Autodesk Inventor part; units mm, degrees
(part 3 of 3)
sketch "Sketch8" plane through (0, 0, 0) normal (0, 0, 1) x (1, 0, 0)
  line L0 (6.1983, 26.6612) -> (5.4238, 26.6612) construction
  line L1 (6.1983, 14.8446) -> (6.1983, 26.6612) projected
  line L2 (6.1293, 14.2121) -> (6.1983, 14.8446) construction
  line L3 (5.9709, 13.7973) -> (6.1293, 14.2121) construction
  line L4 (5.9268, 13.7518) -> (5.9709, 13.7973) construction
  line L5 (5.8813, 13.7077) -> (5.9268, 13.7518) construction
  line L6 (5.4417, 13.5533) -> (5.8813, 13.7077) construction
  line L7 (4.7582, 13.4872) -> (5.4417, 13.5533) construction
  line L8 (3.0618, 13.4872) -> (4.7582, 13.4872) projected
  line L9 (3.0618, 11.5607) -> (3.0618, 13.4872) projected
  line L10 (12.9024, 11.5607) -> (3.0618, 11.5607) projected
  line L11 (12.9024, 13.4872) -> (12.9024, 11.5607) projected
  line L12 (11.2267, 13.4872) -> (12.9024, 13.4872) projected
  line L13 (10.5363, 13.5547) -> (11.2267, 13.4872) construction
  line L14 (10.0898, 13.7132) -> (10.5363, 13.5547) construction
  line L15 (10.0444, 13.7587) -> (10.0898, 13.7132) construction
  line L16 (9.9975, 13.8041) -> (10.0444, 13.7587) construction
  line L17 (9.8349, 14.2189) -> (9.9975, 13.8041) construction
  line L18 (9.766, 14.8473) -> (9.8349, 14.2189) construction
  line L19 (9.766, 26.6612) -> (9.766, 14.8473)
  line L20 (10.5736, 26.6612) -> (9.766, 26.6612) construction
  line L21 (11.8854, 26.3526) -> (10.5736, 26.6612) construction
  line L22 (12.9327, 25.6333) -> (11.8854, 26.3526) construction
  line L23 (13.0871, 25.4265) -> (12.9327, 25.6333) construction
  line L24 (13.2414, 25.2212) -> (13.0871, 25.4265) construction
  line L25 (13.7871, 23.828) -> (13.2414, 25.2212) construction
  line L26 (14.0338, 21.9483) -> (13.7871, 23.828) construction
  line L27 (14.0379, 21.4991) -> (14.0338, 21.9483) construction
  line L28 (15.9768, 21.4991) -> (14.0379, 21.4991)
  line L29 (15.9768, 28.5255) -> (15.9768, 21.4991)
  line L30 (0, 28.5255) -> (15.9768, 28.5255) projected
  line L31 (0, 21.4988) -> (0, 28.5255) projected
  line L32 (1.9389, 21.4988) -> (0, 21.4988) projected
  line L33 (1.9444, 21.9535) -> (1.9389, 21.4988) construction
  line L34 (2.198, 23.8497) -> (1.9444, 21.9535) construction
  line L35 (2.7478, 25.2415) -> (2.198, 23.8497) construction
  line L36 (2.9022, 25.4442) -> (2.7478, 25.2415) construction
  line L37 (3.0565, 25.6467) -> (2.9022, 25.4442) construction
  line L38 (4.1051, 26.3565) -> (3.0565, 25.6467) construction
  line L39 (5.4238, 26.6612) -> (4.1051, 26.3565) construction
  line L40 (1.9444, 21.9535) -> (1.9389, 21.4988) construction
  line L41 (2.198, 23.8497) -> (1.9444, 21.9535) construction
  line L42 (2.7478, 25.2415) -> (2.198, 23.8497) construction
  line L43 (4.1051, 26.3565) -> (3.0565, 25.6467) construction
  line L44 (5.4238, 26.6612) -> (4.1051, 26.3565) construction
  line L45 (6.1983, 26.6612) -> (5.4238, 26.6612) construction
  line L46 (11.8854, 26.3526) -> (10.5736, 26.6612) construction
  line L47 (10.5736, 26.6612) -> (9.766, 26.6612) construction
  line L48 (12.9327, 25.6333) -> (11.8854, 26.3526) construction
  line L49 (13.7871, 23.828) -> (13.2414, 25.2212) construction
  line L50 (14.0338, 21.9483) -> (13.7871, 23.828) construction
  line L51 (14.0379, 21.4991) -> (14.0338, 21.9483) construction
  line L52 (6.1293, 14.2121) -> (6.1983, 14.8446) construction
  line L53 (5.9709, 13.7973) -> (6.1293, 14.2121) construction
  line L54 (5.4417, 13.5533) -> (5.8813, 13.7077) construction
  line L55 (4.7582, 13.4872) -> (5.4417, 13.5533) construction
  line L56 (10.5363, 13.5547) -> (11.2267, 13.4872) construction
  line L57 (10.0898, 13.7132) -> (10.5363, 13.5547) construction
  line L58 (10.0444, 13.7587) -> (10.0898, 13.7132) construction
  line L59 (9.9975, 13.8041) -> (10.0444, 13.7587) construction
  line L60 (9.8349, 14.2189) -> (9.9975, 13.8041) construction
  line L61 (9.766, 14.8473) -> (9.8349, 14.2189) construction
  line L62 (1.9389, 21.4988) -> (0, 21.4988)
  line L63 (1.9389, 21.4988) -> (0, 21.4988) projected
  line L64 (0, 21.4988) -> (0, 28.5255)
  line L65 (15.9768, 28.5255) -> (15.9768, 21.4991)
  line L66 (15.9768, 21.4991) -> (14.0379, 21.4991) projected
  line L67 (15.9768, 21.4991) -> (14.0379, 21.4991)
  line L68 (4.7582, 13.4872) -> (3.0618, 13.4872)
  line L69 (12.9024, 11.5607) -> (3.0618, 11.5607) projected
  line L70 (3.0618, 13.4872) -> (3.0618, 11.5607)
  line L71 (3.0618, 11.5607) -> (12.9024, 11.5607)
  line L72 (12.9024, 13.4872) -> (11.2267, 13.4872)
  line L73 (12.9024, 13.4872) -> (12.9024, 11.5607)
  line L74 (9.766, 26.6612) -> (9.766, 14.8473) projected
  line L75 (9.766, 14.8473) -> (9.766, 26.6612)
  line L76 (6.1983, 26.6612) -> (5.811, 26.6612) construction
  line L77 (5.811, 26.6612) -> (5.4238, 26.6612) construction
  line L78 (5.4238, 26.6612) -> (4.1051, 26.3565) construction
  line L79 (4.1051, 26.3565) -> (3.0565, 25.6467) construction
  line L80 (3.0565, 25.6467) -> (2.9022, 25.4442) construction
  line L81 (2.9022, 25.4442) -> (2.7478, 25.2415) construction
  line L82 (2.7478, 25.2415) -> (2.4729, 24.5456) construction
  line L83 (2.4729, 24.5456) -> (2.198, 23.8497) construction
  line L84 (2.198, 23.8497) -> (2.0712, 22.9016) construction
  line L85 (2.0712, 22.9016) -> (1.9444, 21.9535) construction
  line L86 (1.9444, 21.9535) -> (1.9417, 21.7261) construction
  line L87 (1.9417, 21.7261) -> (1.9389, 21.4988) construction
  spline S0 degree 4 poles (6.1983, 26.6612) (5.811, 26.6612) (5.4238, 26.6612) (4.1051, 26.3565) (3.0565, 25.6467) (2.9022, 25.4442) (2.7478, 25.2415) (2.4729, 24.5456) (2.198, 23.8497) (2.0712, 22.9016) (1.9444, 21.9535) (1.9417, 21.7261) (1.9389, 21.4988) knots 1 1 1 1 1 2 3 4 5 6 7 8 9 10 10 10 10 10
  line L88 (6.1983, 26.6612) -> (6.1983, 14.8446)
  line L89 (9.766, 26.6612) -> (10.1698, 26.6612) construction
  line L90 (10.1698, 26.6612) -> (10.5736, 26.6612) construction
  line L91 (10.5736, 26.6612) -> (11.2295, 26.5069) construction
  line L92 (11.2295, 26.5069) -> (11.8854, 26.3526) construction
  line L93 (11.8854, 26.3526) -> (12.4091, 25.9929) construction
  line L94 (12.4091, 25.9929) -> (12.9327, 25.6333) construction
  line L95 (12.9327, 25.6333) -> (13.0871, 25.4265) construction
  line L96 (13.0871, 25.4265) -> (13.2414, 25.2212) construction
  line L97 (13.2414, 25.2212) -> (13.5143, 24.5246) construction
  line L98 (13.5143, 24.5246) -> (13.7871, 23.828) construction
  line L99 (13.7871, 23.828) -> (13.9105, 22.8882) construction
  line L100 (13.9105, 22.8882) -> (14.0338, 21.9483) construction
  line L101 (14.0338, 21.9483) -> (14.0359, 21.7237) construction
  line L102 (14.0359, 21.7237) -> (14.0379, 21.4991) construction
  spline S1 degree 4 poles (9.766, 26.6612) (10.1698, 26.6612) (10.5736, 26.6612) (11.2295, 26.5069) (11.8854, 26.3526) (12.4091, 25.9929) (12.9327, 25.6333) (13.0871, 25.4265) (13.2414, 25.2212) (13.5143, 24.5246) (13.7871, 23.828) (13.9105, 22.8882) (14.0338, 21.9483) (14.0359, 21.7237) (14.0379, 21.4991) knots 1 1 1 1 1 2 3 4 5 6 7 8 9 10 11 12 12 12 12 12
  line L103 (4.7582, 13.4872) -> (5.1, 13.5203) construction
  line L104 (5.1, 13.5203) -> (5.4417, 13.5533) construction
  line L105 (5.4417, 13.5533) -> (5.6615, 13.6305) construction
  line L106 (5.6615, 13.6305) -> (5.8813, 13.7077) construction
  line L107 (5.8813, 13.7077) -> (5.9268, 13.7518) construction
  line L108 (5.9268, 13.7518) -> (5.9709, 13.7973) construction
  line L109 (5.9709, 13.7973) -> (6.0501, 14.0047) construction
  line L110 (6.0501, 14.0047) -> (6.1293, 14.2121) construction
  line L111 (6.1293, 14.2121) -> (6.1638, 14.5283) construction
  line L112 (6.1638, 14.5283) -> (6.1983, 14.8446) construction
  spline S2 degree 4 poles (4.7582, 13.4872) (5.1, 13.5203) (5.4417, 13.5533) (5.6615, 13.6305) (5.8813, 13.7077) (5.9268, 13.7518) (5.9709, 13.7973) (6.0501, 14.0047) (6.1293, 14.2121) (6.1638, 14.5283) (6.1983, 14.8446) knots 1 1 1 1 1 2 3 4 5 6 7 8 8 8 8 8
  line L113 (9.766, 14.8473) -> (9.8004, 14.5331) construction
  spline S3 degree 4 poles (9.766, 14.8473) (9.8004, 14.5331) (9.8349, 14.2189) (9.9162, 14.0115) (9.9975, 13.8041) (10.0444, 13.7587) (10.0898, 13.7132) (10.3131, 13.634) (10.5363, 13.5547) (10.8815, 13.521) (11.2267, 13.4872) knots 1 1 1 1 1 1.286824 1.330759 1.381504 1.474538 1.728419 1.8309 2 2 2 2 2
  line L114 (10.8815, 13.521) -> (11.2267, 13.4872) construction
  line L115 (10.3131, 13.634) -> (10.5363, 13.5547) construction
  line L116 (10.5363, 13.5547) -> (10.8815, 13.521) construction
  line L117 (10.0444, 13.7587) -> (10.0898, 13.7132) construction
  line L118 (10.0898, 13.7132) -> (10.3131, 13.634) construction
  line L119 (9.8004, 14.5331) -> (9.8349, 14.2189) construction
  line L120 (9.8349, 14.2189) -> (9.9162, 14.0115) construction
  line L121 (9.9162, 14.0115) -> (9.9975, 13.8041) construction
  line L122 (9.9975, 13.8041) -> (10.0444, 13.7587) construction
  line L123 (9.766, 26.6612) -> (9.766, 14.8473)
  line L124 (1.9389, 21.4988) -> (0, 21.4988)
  line L125 (0, 21.4988) -> (0, 28.5255)
  line L126 (14.0379, 21.4991) -> (15.9768, 21.4991)
  line L127 (15.9768, 21.4991) -> (15.9768, 28.5255)
  line L128 (4.7582, 13.4872) -> (3.0618, 13.4872)
  line L129 (3.0618, 11.5607) -> (3.0618, 13.4872) projected
  line L130 (3.0618, 13.4872) -> (3.0618, 11.5607)
  line L131 (3.0618, 11.5607) -> (12.9024, 11.5607)
  line L132 (12.9024, 13.4872) -> (12.9024, 11.5607) projected
  line L133 (12.9024, 11.5607) -> (12.9024, 13.4872)
  line L134 (12.9024, 13.4872) -> (11.2267, 13.4872)
  line L135 (9.766, 26.6612) -> (9.766, 14.8473) projected
  line L136 (9.766, 14.8473) -> (9.766, 26.6612)
  line L137 (6.1983, 14.8446) -> (6.1983, 26.6612) projected
  line L138 (6.1983, 26.6612) -> (6.1983, 14.8446)
  line L139 (0, 28.5255) -> (15.9768, 28.5255) projected
  line L140 (15.9768, 28.5255) -> (0, 28.5255)
  line L141 (0, 21.4988) -> (0, 28.5255) projected
  line L142 (0, 28.5255) -> (0, 21.4988)
  line L143 (0, 21.4988) -> (1.9389, 21.4988)
  point P0 (0, 0)
  point P1 (1.9417, 21.7261)
  point P2 (1.9444, 21.9535)
  point P3 (2.0712, 22.9016)
  point P4 (2.4729, 24.5456)
  point P5 (11.2295, 26.5069)
  point P6 (12.4091, 25.9929)
  point P7 (14.0359, 21.7237)
  point P8 (9.8004, 14.5331)
  point P9 (1.9417, 21.7261)
  point P10 (2.0712, 22.9016)
  point P11 (2.4729, 24.5456)
  point P12 (11.2295, 26.5069)
  point P13 (14.0359, 21.7237)
  point P14 (12.4091, 25.9929)
  point P15 (9.8004, 14.5331)
  constraints: 71 coincident, 58 end point, 31 midpoint, 15 point on line, 11 collinear, 5 horizontal, 5 perpendicular, 4 vertical, 17 other
sketch "Sketch9" plane through (0, 0, 0) normal (0, 0, 1) x (1, 0, 0)
  line L0 (0, 28.5255) -> (15.9768, 28.5255)
  line L1 (15.9768, 28.5255) -> (15.9768, 11.5607)
  line L2 (15.9768, 11.5607) -> (0, 11.5607)
  line L3 (0, 11.5607) -> (0, 28.5255)
  line L4 (12.9024, 11.5607) -> (3.0618, 11.5607) projected
  point P0 (0, 0)
  point P1 (15.9768, 21.4991)
  constraints: 8 end point, 2 parallel, 2 point on line, 1 horizontal, 1 perpendicular
extrude "Extrusion6" cut sketch "Sketch9" against normal through all
extrude "Extrusion7" add sketch "Sketch8" against normal blind 25.4
sketch "Sketch10" plane through (0, 0, 0) normal (0, 0, 1) x (1, 0, 0)
  line L0 (4.7582, 13.4872) -> (3.0618, 13.4872) projected
  line L1 (3.0618, 13.4872) -> (3.0618, 11.5607) projected
  line L2 (3.0618, 11.5607) -> (12.9024, 11.5607) projected
  line L3 (12.9024, 11.5607) -> (12.9024, 13.4872) projected
  line L4 (12.9024, 13.4872) -> (11.2267, 13.4872) projected
  line L5 (9.766, 14.8473) -> (9.766, 26.6612) projected
  line L6 (14.0379, 21.4991) -> (15.9768, 21.4991) projected
  line L7 (15.9768, 21.4991) -> (15.9768, 28.5255) projected
  line L8 (15.9768, 28.5255) -> (0, 28.5255) projected
  line L9 (0, 28.5255) -> (0, 21.4988) projected
  line L10 (0, 21.4988) -> (1.9389, 21.4988) projected
  line L11 (6.1983, 26.6612) -> (6.1983, 14.8446) projected
  spline S0 degree 4 poles (45.6766, 1.7915) (45.6619, 1.6499) (45.6472, 1.5084) (45.6123, 1.4155) (45.5774, 1.3225) (45.5577, 1.3021) (45.5375, 1.2822) (45.4394, 1.2472) (45.3413, 1.2122) (45.1885, 1.1966) (45.0357, 1.181) knots 1 1 1 1 1 2 3 4 5 6 7 8 8 8 8 8
  line L12 (45.0357, 1.181) -> (44.1536, 1.181)
  line L13 (44.1536, 1.181) -> (44.1536, 0.2453)
  line L14 (44.1536, 0.2453) -> (48.9313, 0.2453)
  line L15 (48.9313, 0.2453) -> (48.9313, 1.181)
  line L16 (48.9313, 1.181) -> (48.0631, 1.181)
  spline S1 degree 4 poles (48.0631, 1.181) (47.909, 1.1955) (47.7548, 1.2101) (47.655, 1.2451) (47.5552, 1.2801) (47.5348, 1.3003) (47.5138, 1.3206) (47.4772, 1.413) (47.4406, 1.5055) (47.4247, 1.6457) (47.4088, 1.7859) knots 1 1 1 1 1 1.1691 1.271581 1.525462 1.618496 1.669241 1.713176 2 2 2 2 2
  line L17 (47.4088, 1.7859) -> (47.4088, 7.5792)
  spline S2 degree 4 poles (47.4088, 7.5792) (47.6049, 7.5792) (47.8011, 7.5793) (48.1196, 7.5044) (48.4382, 7.4295) (48.6926, 7.2549) (48.9469, 7.0803) (49.0219, 6.9799) (49.0969, 6.8802) (49.2294, 6.5419) (49.362, 6.2036) (49.422, 5.7472) (49.482, 5.2907) (49.483, 5.1816) (49.484, 5.0726) knots 1 1 1 1 1 2 3 4 5 6 7 8 9 10 11 12 12 12 12 12
  line L18 (49.484, 5.0726) -> (50.4254, 5.0726)
  line L19 (50.4254, 5.0726) -> (50.4254, 8.4846)
  line L20 (50.4254, 8.4846) -> (42.6667, 8.4846)
  line L21 (42.6667, 8.4846) -> (42.6667, 5.0726)
  line L22 (42.6667, 5.0726) -> (43.608, 5.0726)
  spline S3 degree 4 poles (43.608, 5.0726) (43.6093, 5.183) (43.6107, 5.2934) (43.6723, 5.7538) (43.7339, 6.2142) (43.8674, 6.5521) (44.001, 6.89) (44.0759, 6.9884) (44.1509, 7.0867) (44.6601, 7.4313) (45.3005, 7.5792) (45.4885, 7.5792) (45.6766, 7.5792) knots 1 1 1 1 1 2 3 4 5 6 7 8 9 10 10 10 10 10
  line L23 (45.6766, 7.5792) -> (45.6766, 1.7915)
  line L24 (42.6667, 8.4846) -> (50.4254, 8.4846) projected
  line L25 (45.6766, 1.7915) -> (45.6766, 7.5792) projected
  line L26 (46.546, 8.4846) -> (46.546, 5.9446) construction
  point P0 (0, 0)
  point P1 (44.1536, 0.2453)
  dimension "d26" = 2.54
  constraints: 26 end point, 10 coincident, 2 midpoint, 1 collinear, 1 vertical, 13 other
  measures "d26" distance of L26.start L26.end
sketch "Sketch11" plane through (0, 0, 0) normal (0, 0, 1) x (1, 0, 0)
  line L0 (41.274, 9.5972) -> (51.7266, 9.5972)
  line L1 (51.7266, 9.5972) -> (51.7266, -1.4993)
  line L2 (51.7266, -1.4993) -> (41.274, -1.4993)
  line L3 (41.274, -1.4993) -> (41.274, 9.5972)
  line L4 (42.6667, 8.4846) -> (50.4254, 8.4846) projected
  line L5 (42.6667, 5.0726) -> (42.6667, 8.4846) projected
  line L6 (48.9313, 0.2453) -> (44.1536, 0.2453) projected
  line L7 (50.4254, 8.4846) -> (50.4254, 5.0726) projected
  point P0 (0, 0)
  dimension "d27" = 1.1126
  dimension "d28" = 1.3927
  dimension "d29" = 1.7446
  dimension "d30" = 1.3013
  constraints: 8 end point, 2 parallel, 1 horizontal, 1 perpendicular
  measures "d27" distance between parallel lines of L0 L4
  measures "d28" distance between parallel lines of L3 L5
  measures "d29" distance between parallel lines of L2 L6
  measures "d30" distance between parallel lines of L1 L7
extrude "Extrusion8" cut sketch "Sketch11" against normal through all
extrude "Extrusion9" add sketch "Sketch10" against normal blind 25.4
sketch "Sketch12" plane through (0, 0, 0) normal (0, 0, 1) x (1, 0, 0)
  line L0 (69.1459, 3.4353) -> (70.2, 3.4353) construction
  line L1 (69.1154, 3.2479) -> (69.1459, 3.4353) construction
  line L2 (68.8688, 2.4431) -> (69.1154, 3.2479) construction
  line L3 (68.4954, 1.8175) -> (68.8688, 2.4431) construction
  line L4 (68.4019, 1.7183) -> (68.4954, 1.8175) construction
  line L5 (68.3067, 1.6204) -> (68.4019, 1.7183) construction
  line L6 (67.7512, 1.2759) -> (68.3067, 1.6204) construction
  line L7 (67.1367, 1.1271) -> (67.7512, 1.2759) construction
  line L8 (66.6734, 1.1271) -> (67.1367, 1.1271) construction
  line L9 (65.8992, 1.3352) -> (66.6734, 1.1271) construction
  line L10 (65.2335, 1.8203) -> (65.8992, 1.3352) construction
  line L11 (65.1273, 1.9581) -> (65.2335, 1.8203) construction
  line L12 (65.0202, 2.0972) -> (65.1273, 1.9581) construction
  line L13 (64.6465, 2.9613) -> (65.0202, 2.0972) construction
  line L14 (64.4867, 3.9741) -> (64.6465, 2.9613) construction
  line L15 (64.4867, 4.6673) -> (64.4867, 3.9741) construction
  line L16 (64.6478, 5.738) -> (64.4867, 4.6673) construction
  line L17 (65.0239, 6.6668) -> (64.6478, 5.738) construction
  line L18 (65.1316, 6.817) -> (65.0239, 6.6668) construction
  line L19 (65.2378, 6.9686) -> (65.1316, 6.817) construction
  line L20 (65.8977, 7.4964) -> (65.2378, 6.9686) construction
  line L21 (66.6556, 7.7224) -> (65.8977, 7.4964) construction
  line L22 (67.1283, 7.7224) -> (66.6556, 7.7224) construction
  line L23 (67.7897, 7.5612) -> (67.1283, 7.7224) construction
  line L24 (68.3905, 7.1836) -> (67.7897, 7.5612) construction
  line L25 (68.4938, 7.0747) -> (68.3905, 7.1836) construction
  line L26 (68.5959, 6.9672) -> (68.4938, 7.0747) construction
  line L27 (68.9912, 6.2948) -> (68.5959, 6.9672) construction
  line L28 (69.2284, 5.4431) -> (68.9912, 6.2948) construction
  line L29 (69.2533, 5.2461) -> (69.2284, 5.4431) construction
  line L30 (70.2, 5.2461) -> (69.2533, 5.2461) construction
  line L31 (70.2, 8.6224) -> (70.2, 5.2461) construction
  line L32 (69.3128, 8.6224) -> (70.2, 8.6224) construction
  line L33 (69.0672, 7.8852) -> (69.3128, 8.6224) construction
  line L34 (68.9737, 7.9568) -> (69.0672, 7.8852) construction
  line L35 (68.0159, 8.4887) -> (68.9737, 7.9568) construction
  line L36 (67.9193, 8.5232) -> (68.0159, 8.4887) construction
  line L37 (67.8216, 8.5576) -> (67.9193, 8.5232) construction
  line L38 (66.9851, 8.7299) -> (67.8216, 8.5576) construction
  line L39 (66.3179, 8.7299) -> (66.9851, 8.7299) construction
  line L40 (65.2473, 8.4832) -> (66.3179, 8.7299) construction
  line L41 (65.1274, 8.4336) -> (65.2473, 8.4832) construction
  line L42 (65.0075, 8.384) -> (65.1274, 8.4336) construction
  line L43 (63.9229, 7.6522) -> (65.0075, 8.384) construction
  line L44 (63.8266, 7.5544) -> (63.9229, 7.6522) construction
  line L45 (63.7192, 7.4483) -> (63.8266, 7.5544) construction
  line L46 (62.9196, 6.2522) -> (63.7192, 7.4483) construction
  line L47 (62.8675, 6.1185) -> (62.9196, 6.2522) construction
  line L48 (62.8139, 5.9862) -> (62.8675, 6.1185) construction
  line L49 (62.5508, 4.808) -> (62.8139, 5.9862) construction
  line L50 (62.5508, 3.9632) -> (62.5508, 4.808) construction
  line L51 (62.8221, 2.7368) -> (62.5508, 3.9632) construction
  line L52 (62.8769, 2.599) -> (62.8221, 2.7368) construction
  line L53 (62.931, 2.4626) -> (62.8769, 2.599) construction
  line L54 (63.7329, 1.2513) -> (62.931, 2.4626) construction
  line L55 (63.8391, 1.1451) -> (63.7329, 1.2513) construction
  line L56 (63.9338, 1.0487) -> (63.8391, 1.1451) construction
  line L57 (65.0225, 0.3294) -> (63.9338, 1.0487) construction
  line L58 (65.1454, 0.2825) -> (65.0225, 0.3294) construction
  line L59 (65.2668, 0.2356) -> (65.1454, 0.2825) construction
  line L60 (66.3735, 0) -> (65.2668, 0.2356) construction
  line L61 (67.1215, 0) -> (66.3735, 0) construction
  line L62 (68.1426, 0.2246) -> (67.1215, 0) construction
  line L63 (69.041, 0.7469) -> (68.1426, 0.2246) construction
  line L64 (69.1899, 0.8957) -> (69.041, 0.7469) construction
  line L65 (69.3375, 1.0459) -> (69.1899, 0.8957) construction
  line L66 (69.8872, 1.9801) -> (69.3375, 1.0459) construction
  line L67 (70.1798, 3.1625) -> (69.8872, 1.9801) construction
  line L68 (70.2, 3.4353) -> (70.1798, 3.1625) construction
  line L69 (69.2533, 5.2461) -> (70.2, 5.2461)
  line L70 (70.2, 5.2461) -> (70.2, 8.6224)
  line L71 (70.2, 8.6224) -> (69.3128, 8.6224)
  line L72 (69.3128, 8.6224) -> (70.2, 8.6224) projected
  line L73 (69.0672, 7.8852) -> (69.3128, 8.6224) projected
  line L74 (69.3128, 8.6224) -> (69.0672, 7.8852)
  line L75 (69.1459, 3.4353) -> (70.2, 3.4353) projected
  line L76 (69.1459, 3.4353) -> (70.2, 3.4353)
  line L77 (68.9737, 7.9568) -> (69.0672, 7.8852) projected
  spline S0 degree 3 poles (69.0672, 7.8852) (69.036, 7.909) (68.717, 8.1575) (68.2958, 8.3914) (67.6187, 8.6315) (67.0491, 8.7502) (66.1722, 8.7491) (65.5047, 8.5922) (64.6832, 8.2537) (64.1603, 7.895) (63.4468, 7.1792) (63.057, 6.6109) (62.6988, 5.7017) (62.5245, 4.9311) (62.5264, 3.8239) (62.7017, 3.0336) (63.0692, 2.1024) (63.4576, 1.5255) (64.1699, 0.805) (64.6962, 0.4494) (65.5369, 0.1305) (66.2439, -0.0209) (67.2224, -0.0215) (68.1576, 0.1725) (68.9032, 0.5911) (69.5017, 1.1969) (69.9512, 2.0038) (70.1653, 2.8478) (70.1933, 3.3444) (70.2, 3.4353) knots 0 0 0 0 0.011778 0.121339 0.141956 0.227353 0.294079 0.403945 0.429895 0.560729 0.589554 0.73343 0.762049 0.882777 0.96725 1.09286 1.122368 1.267635 1.296166 1.426649 1.452819 1.565968 1.640771 1.74532 1.849238 1.891343 1.999743 2.121541 2.1489 2.1489 2.1489 2.1489
  line L78 (70.2, 3.4353) -> (70.1798, 3.1625) projected
  point P0 (0, 0)
  constraints: 10 end point, 4 collinear, 1 perpendicular, 30 other
body "Solid1"
